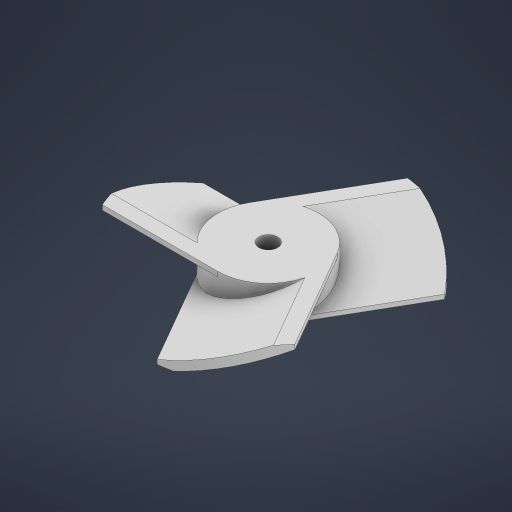
# Autodesk Inventor part: Propeler V.1
Saved by Autodesk Inventor 2024.4 (Build 284460030, 460C)
## iProperties
Created: 2026-08-01
Part Number: Propeler V.1
Material: Generic
Document SubType Name: Modeling
Designer: yulis
Density: 1 g/cm^3
Appearance: Default
Author: yulis
Autodesk Inventor part; units mm, degrees
ref_plane "YZ Plane" through (0, 0, 0) normal (1, 0, 0) x (0, 1, 0)
ref_plane "XZ Plane" through (0, 0, 0) normal (0, 1, 0) x (-1, 0, 0)
ref_plane "XY Plane" through (0, 0, 0) normal (0, 0, 1) x (1, 0, 0)
sketch "Sketch1" plane through (0, 0, 0) normal (0, 1, 0) x (-1, 0, 0)
  circle A0 centre (0, 0) radius 35
  circle A1 centre (0, 0) radius 14
  dimension "d0" = 70
  dimension "d1" = 28
  constraints: 2 centre point, 2 coincident
  measures "d0" diameter of A0
  measures "d1" diameter of A1
extrude "Extrusion1" add sketch "Sketch1" along normal blind 10 contours A1
sketch "Sketch2" plane through (0, 0, 0) normal (1, 0, 0) x (0, 1, 0)
  line L0 (0, 10.0246) -> (8.7928, -14)
  line L1 (10, -10.2835) -> (1.3273, 14)
  line L2 (10, -14) -> (0, -14)
  line L3 (0, 14) -> (10, 14) projected
  line L4 (10, 14) -> (0, 14)
  line L5 (10, -14) -> (10, 14)
  line L6 (0, -14) -> (0, 14) projected
  line L7 (0, -14) -> (0, 14)
  line L8 (10, -10.2835) -> (10, -14)
  line L9 (1.3273, 14) -> (0, 14)
  line L10 (0, 10.0246) -> (0, 14)
  line L11 (0, 14) -> (1.3273, 14)
  point P0 (0, 0)
  point P1 (5, 0)
  constraints: 20 end point, 5 point on line, 2 horizontal, 2 perpendicular, 2 vertical, 1 collinear
extrude "Extrusion2" add sketch "Sketch2" against normal blind 35 contours L6 L3 L1 L5 L2 L0
pattern_circular "Circular Pattern1" count 3 over 360 about axis through (0, 0, 0) along (0, 1, 0) of "Extrusion2"
sketch "Sketch3" plane through (0, 10, 0) normal (0, 1, 0) x (1, 0, 0)
  circle A0 centre (0, 0) radius 35
  dimension "d14" = 70
  constraints: 1 centre point, 1 coincident
  measures "d14" diameter of A0
extrude "Extrusion3" cut sketch "Sketch3" against normal blind 35 keep common part
sketch "Sketch4" plane through (0, 10, 0) normal (0, 1, 0) x (1, 0, 0)
  circle A0 centre (0, 0) radius 2.6
  dimension "d17" = 5.2
  constraints: 1 centre point, 1 coincident
  measures "d17" diameter of A0
extrude "Extrusion4" cut sketch "Sketch4" against normal blind 35
mirror "Mirror1" about plane through (0, 0, 0) normal (0, 1, 0) remove original yes
body "Solid1"
